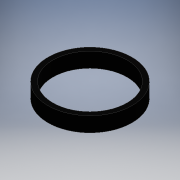
# Autodesk Inventor part: オイレス　15-17
Saved by Autodesk Inventor 2016 (Build 200138000, 138)
## iProperties
Created: 2018-03-17
Part Number: オイレス　15-17
Material: アセタール樹脂、黒
Document SubType Name: Modeling
Designer: Takumi
Density: 1.425 g/cm^3
Appearance: 滑らか - 黒
Mass: 0.214885 g
Surface Area: 4.02124 cm^2
Volume: 0.150796 cm^3
Author: Takumi
Autodesk Inventor part; units mm, degrees
ref_plane "YZ Plane" through (0, 0, 0) normal (1, 0, 0) x (0, 1, 0)
ref_plane "XZ Plane" through (0, 0, 0) normal (0, 1, 0) x (-1, 0, 0)
ref_plane "XY Plane" through (0, 0, 0) normal (0, 0, 1) x (1, 0, 0)
sketch "スケッチ1" plane through (0, 0, 0) normal (0, 0, 1) x (1, 0, 0)
  circle A0 centre (0, 0) radius 7.5
  circle A1 centre (0, 0) radius 8.5
  dimension "d0" = 15
  dimension "d1" = 17
  constraints: 2 centre point, 2 coincident
  measures "d0" diameter of A0
  measures "d1" diameter of A1
extrude "押し出し1" add sketch "スケッチ1" along normal blind 3
